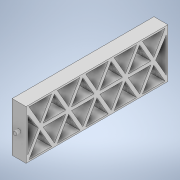
# Autodesk Inventor part: Arm support for bottom arms
Saved by Autodesk Inventor 2020.2 (Build 242310000, 310)
## iProperties
Created: 2020-03-31
Part Number: Arm support for bottom arms
Material: Generic
Document SubType Name: Modeling
Designer: Amaan Khalid
Density: 1 g/cm^3
Appearance: Default
Author: Amaan Khalid
Autodesk Inventor part; units mm, degrees
ref_plane "YZ Plane" through (0, 0, 0) normal (1, 0, 0) x (0, 1, 0)
ref_plane "XZ Plane" through (0, 0, 0) normal (0, 1, 0) x (-1, 0, 0)
ref_plane "XY Plane" through (0, 0, 0) normal (0, 0, 1) x (1, 0, 0)
sketch "Sketch1" plane through (0, 0, 0) normal (1, 0, 0) x (0, 1, 0)
  line L0 (31.4399, 11.0097) -> (31.4399, -9.3256)
  line L1 (31.4399, -9.3256) -> (49.0507, 0.842)
  line L2 (49.0507, 0.842) -> (31.4399, 11.0097)
  line L3 (46.6123, 0.842) -> (32.6591, -7.2139)
  line L4 (32.6591, -7.2139) -> (32.6591, 8.8979)
  line L5 (32.6591, 8.8979) -> (46.6123, 0.842)
  line L6 (49.0507, 0.842) -> (31.4399, -9.3256)
  line L7 (49.0507, -19.4932) -> (31.4399, -9.3256)
  line L8 (49.0507, 0.842) -> (49.0507, -19.4932)
  line L9 (47.8315, -1.2697) -> (33.8783, -9.3256)
  line L10 (33.8783, -9.3256) -> (47.8315, -17.3815)
  line L11 (47.8315, -17.3815) -> (47.8315, -1.2697)
  line L12 (31.4399, -9.3256) -> (31.4399, -29.6608)
  line L13 (31.4399, -29.6608) -> (49.0507, -19.4932)
  line L14 (32.6591, -27.5491) -> (32.6591, -11.4373)
  line L15 (32.6591, -11.4373) -> (46.6123, -19.4932)
  line L16 (46.6123, -19.4932) -> (32.6591, -27.5491)
  line L17 (49.0507, -19.4932) -> (49.0507, -39.8284)
  line L18 (49.0507, -39.8284) -> (31.4399, -29.6608)
  line L19 (47.8315, -37.7167) -> (47.8315, -21.6049)
  line L20 (33.8783, -29.6608) -> (47.8315, -37.7167)
  line L21 (47.8315, -21.6049) -> (33.8783, -29.6608)
  line L22 (31.4399, -29.6608) -> (31.4399, -49.9961)
  line L23 (32.6591, -47.8843) -> (32.6591, -31.7725)
  line L24 (31.4399, -49.9961) -> (49.0507, -39.8284)
  line L25 (46.6123, -39.8284) -> (32.6591, -47.8843)
  line L26 (32.6591, -31.7725) -> (46.6123, -39.8284)
  line L27 (49.0507, -39.8284) -> (49.0507, -60.1637)
  line L28 (47.8315, -41.9402) -> (33.8783, -49.9961)
  line L29 (33.8783, -49.9961) -> (47.8315, -58.052)
  line L30 (49.0507, -60.1637) -> (31.4399, -49.9961)
  line L31 (47.8315, -58.052) -> (47.8315, -41.9402)
  line L32 (31.4399, -49.9961) -> (31.4399, -70.3313)
  line L33 (31.4399, -70.3313) -> (49.0507, -60.1637)
  line L34 (46.6123, -60.1637) -> (32.6591, -68.2196)
  line L35 (32.6591, -68.2196) -> (32.6591, -52.1078)
  line L36 (32.6591, -52.1078) -> (46.6123, -60.1637)
  line L37 (31.4399, -9.3256) -> (13.8291, 0.842)
  line L38 (13.8291, 0.842) -> (31.4399, 11.0097)
  line L39 (16.2675, 0.842) -> (30.2207, -7.2139)
  line L40 (30.2207, -7.2139) -> (30.2207, 8.8979)
  line L41 (30.2207, 8.8979) -> (16.2675, 0.842)
  line L42 (31.4399, -9.3256) -> (13.8291, 0.842)
  line L43 (13.8291, -19.4932) -> (31.4399, -9.3256)
  line L44 (13.8291, 0.842) -> (13.8291, -19.4932)
  line L45 (15.0483, -1.2697) -> (29.0015, -9.3256)
  line L46 (29.0015, -9.3256) -> (15.0483, -17.3815)
  line L47 (15.0483, -17.3815) -> (15.0483, -1.2697)
  line L48 (13.8291, -19.4932) -> (31.4399, -9.3256)
  line L49 (31.4399, -29.6608) -> (13.8291, -19.4932)
  line L50 (30.2207, -11.4373) -> (16.2675, -19.4932)
  line L51 (30.2207, -27.5491) -> (30.2207, -11.4373)
  line L52 (16.2675, -19.4932) -> (30.2207, -27.5491)
  line L53 (13.8291, -39.8284) -> (31.4399, -29.6608)
  line L54 (16.2675, -39.8284) -> (30.2207, -47.8843)
  line L55 (30.2207, -47.8843) -> (30.2207, -31.7725)
  line L56 (31.4399, -49.9961) -> (13.8291, -39.8284)
  line L57 (30.2207, -31.7725) -> (16.2675, -39.8284)
  line L58 (31.4399, -29.6608) -> (13.8291, -19.4932)
  line L59 (15.0483, -21.6049) -> (29.0015, -29.6608)
  line L60 (13.8291, -19.4932) -> (13.8291, -39.8284)
  line L61 (15.0483, -37.7167) -> (15.0483, -21.6049)
  line L62 (13.8291, -39.8284) -> (31.4399, -29.6608)
  line L63 (29.0015, -29.6608) -> (15.0483, -37.7167)
  line L64 (13.8291, -60.1637) -> (31.4399, -49.9961)
  line L65 (30.2207, -68.2196) -> (30.2207, -52.1078)
  line L66 (31.4399, -70.3313) -> (13.8291, -60.1637)
  line L67 (30.2207, -52.1078) -> (16.2675, -60.1637)
  line L68 (16.2675, -60.1637) -> (30.2207, -68.2196)
  line L69 (31.4399, -49.9961) -> (13.8291, -39.8284)
  line L70 (13.8291, -39.8284) -> (13.8291, -60.1637)
  line L71 (15.0483, -58.052) -> (15.0483, -41.9402)
  line L72 (15.0483, -41.9402) -> (29.0015, -49.9961)
  line L73 (13.8291, -60.1637) -> (31.4399, -49.9961)
  line L74 (29.0015, -49.9961) -> (15.0483, -58.052)
  line L75 (13.8291, 0.842) -> (13.8291, 21.1773)
  line L76 (13.8291, 21.1773) -> (31.4399, 11.0097)
  line L77 (49.0507, 0.842) -> (49.0507, 21.1773)
  line L78 (49.0507, 21.1773) -> (31.4399, 11.0097)
  line L79 (49.0507, 21.1773) -> (13.8291, 21.1773)
  line L80 (49.0507, -60.1637) -> (49.0507, -80.4989)
  line L81 (49.0507, -80.4989) -> (31.4399, -70.3313)
  line L82 (13.8291, -60.1637) -> (13.8291, -80.4989)
  line L83 (13.8291, -80.4989) -> (31.4399, -70.3313)
  line L84 (49.0507, -80.4989) -> (13.8291, -80.4989)
  line L85 (15.0483, 2.9538) -> (15.0483, 19.0656)
  line L86 (29.0015, 11.0097) -> (15.0483, 2.9538)
  line L87 (15.0483, 19.0656) -> (29.0015, 11.0097)
  line L88 (47.8315, 2.9538) -> (47.8315, 19.0656)
  line L89 (47.8315, 19.0656) -> (33.8783, 11.0097)
  line L90 (33.8783, 11.0097) -> (47.8315, 2.9538)
  line L91 (33.8783, -70.3313) -> (47.8315, -78.3872)
  line L92 (47.8315, -78.3872) -> (47.8315, -62.2754)
  line L93 (47.8315, -62.2754) -> (33.8783, -70.3313)
  line L94 (29.0015, -70.3313) -> (15.0483, -78.3872)
  line L95 (15.0483, -78.3872) -> (15.0483, -62.2754)
  line L96 (15.0483, -62.2754) -> (29.0015, -70.3313)
  line L97 (33.4035, 19.9572) -> (43.2391, 19.9572)
  line L98 (43.2391, 19.9572) -> (31.4399, 12.4185)
  line L99 (31.4399, 12.4185) -> (18.3826, 19.9572)
  line L100 (18.3826, 19.9572) -> (33.4035, 19.9572)
  line L101 (33.4035, -79.2788) -> (43.2391, -79.2788)
  line L102 (43.2391, -79.2788) -> (31.4399, -71.7402)
  line L103 (31.4399, -71.7402) -> (18.3826, -79.2788)
  line L104 (18.3826, -79.2788) -> (33.4035, -79.2788)
  dimension "d13" = 1.2192
  constraints: 210 end point, 61 symmetric about line, 5 vertical, 3 collinear, 2 point on line, 1 parallel, 2 other
  measures "d13" distance between parallel lines of L1 L3
extrude "Extrusion1" add sketch "Sketch1" along normal blind 10
sketch "Sketch2" plane through (0, 13.8291, 21.1773) normal (0, 0, 1) x (1, 0, 0)
  line L0 (0, 35.2217) -> (10, 35.2217) projected
  circle A0 centre (5.0038, 17.6108) radius 1.27
  point P0 (0, -13.8291)
  point P1 (0, 17.6108)
  constraints: 1 centre point
extrude "Extrusion2" add sketch "Sketch2" along normal blind 3
sketch "Sketch3" plane through (0, 13.8291, -80.4989) normal (0, 0, -1) x (-1, 0, 0)
  line L0 (0, 35.2217) -> (-10, 35.2217) projected
  line L1 (0, 18.83) -> (-10, 18.83) projected
  circle A0 centre (-5, 18.83) radius 1.27
  point P0 (0, -13.8291)
  dimension "d36" = 2.54
  constraints: 1 centre point, 1 midpoint
  measures "d36" diameter of A0
extrude "Extrusion3" add sketch "Sketch3" along normal blind 3
body "Solid1"
